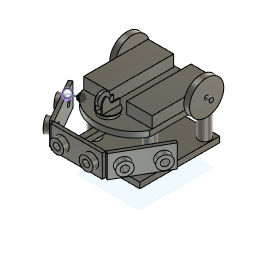
Chassis v4 (Autodesk Fusion 360 design; units mm, degrees)
Autodesk Fusion 360 part; units mm, degrees
sketch "Sketch1" plane through (0, 0, 0) normal (1, 0, 0) x (0, 1, 0)
  line L0 (30, -30) -> (-30, -30)
  line L1 (-30, -30) -> (-30, 30)
  line L2 (30, 30) -> (30, -30)
  line L3 (30, -30) -> (-30, 30) construction
  line L4 (-30, -30) -> (30, 30) construction
  arc A0 (30, 30) -> (-30, 30) centre (0, 12.4031) ccw
  dimension "d1" = 60
  dimension "d2" = 60
  constraint horizontal L0
  constraint perpendicular L0 L1
  constraint parallel L1 L2
  constraint coincident L3 origin
  constraint coincident L4 origin
  measures "d1" distance of L1.end L2.start
  measures "d2" distance of L0.end L1.end
extrude "Extrude1" add sketch "Sketch1" along normal blind 5 makes body 1
move_body "Move1" bodies 1 to x (0, 0, 1) y (-1, 0, 0) z (0, -1, 0) at (-30, -60, 0)
sketch "Sketch2" plane through (0, 0, 0) normal (0, 0, -1) x (1, 0, 0)
  line L0 (-60, 90) -> (-60, 30)
  line L1 (-60, 30) -> (0, 30)
  line L2 (0, 30) -> (0, 90)
  arc A0 (0, 90) -> (-60, 90) centre (-30, 72.4031) ccw
  circle A1 centre (-5.7984, 36.1081) radius 5
  line L3 (-30, 27.885) -> (-30, 109.1678) construction
  line L4 (-30, 27.885) -> (-30, 109.1678) construction
  circle A2 centre (-54.2016, 36.1081) radius 5
  line L5 (25, 60) -> (-75, 60) construction
  line L6 (25, 60) -> (-75, 60) construction
  circle A3 centre (-5.7984, 83.8919) radius 5
  circle A4 centre (-54.2016, 83.8919) radius 5
  dimension "d5" = 10
  constraint perpendicular L1 L3
  constraint symmetric A1 L3 A2
  constraint symmetric L4.start L3 L3.start
  constraint symmetric L4.end L3 L3.end
  constraint perpendicular L0 L5
  constraint symmetric A1 L5 A3
  constraint symmetric A2 L5 A4
  constraint symmetric L6.start L5 L5.start
  constraint symmetric L6.end L5 L5.end
  measures "d5" diameter of A1
extrude "Extrude2" add sketch "Sketch2" along normal blind 30 contours A1 | A2 | A3 | A4 bodies 1
ref_plane "WorkPlane1" through (-30, -68.5916, -50) normal (0, 0, -1) x (1, 0, 0)
sketch "Sketch3" plane through (-30, -68.5916, -50) normal (0, 0, -1) x (-1, 0, 0)
  line L0 (-30, -21.4084) -> (-30, 38.5916)
  line L1 (30, 38.5916) -> (30, -21.4084)
  line L2 (-30, -30) -> (-30, 40)
  line L3 (30, 40) -> (-30, 40)
  line L4 (-30, -30) -> (30, -30)
  line L5 (30, -30) -> (30, 40)
  point P0 (-30, 38.5916)
  point P1 (30, 38.5916)
  point P2 (30, -21.4084)
  point P3 (-30, -21.4084)
  dimension "d10" = 60
  dimension "d11" = 70
  constraint vertical L0
  constraint vertical L1
  constraint coincident P0 L0.end
  constraint coincident P2 L1.end
  constraint perpendicular L2 L3
  constraint perpendicular L2 L4
  constraint perpendicular L3 L5
  measures "d10" distance of P2 P3
  measures "d11" distance of L2.start L2.end
extrude "Extrude3" add sketch "Sketch3" along normal blind 5 bodies 1 makes body 2
sketch "Sketch4" plane through (0, 0, 5) normal (0, 0, 1) x (-1, 0, 0)
  line L0 (60, 30) -> (60, 90)
  arc A0 (60, 90) -> (0, 90) centre (30, 72.4031) ccw
  line L1 (0, 90) -> (0, 30)
  line L2 (0, 30) -> (60, 30)
  line L3 (0, 87.7947) -> (22.4, 87.7947)
  line L4 (22.4, 87.7947) -> (22.4, 31.2947)
  line L5 (22.4, 31.2947) -> (0, 31.2947)
  line L6 (0, 31.2947) -> (0, 87.7947)
  line L7 (30, 125) -> (30, 18.4359) construction
  line L8 (30, 125) -> (30, 18.4359) construction
  line L9 (60, 87.7947) -> (37.6, 87.7947)
  line L10 (37.6, 87.7947) -> (37.6, 31.2947)
  line L11 (37.6, 31.2947) -> (60, 31.2947)
  line L12 (60, 31.2947) -> (60, 87.7947)
  dimension "d14" = 22.4
  dimension "d15" = 56.5
  constraint horizontal L3
  constraint vertical L4
  constraint horizontal L5
  constraint vertical L6
  constraint coincident L1 L3.start
  constraint perpendicular L2 L7
  constraint symmetric L3.start L7 L9.start
  constraint symmetric L3.end L7 L9.end
  constraint symmetric L4.end L7 L10.end
  constraint symmetric L5.end L7 L11.end
  constraint symmetric L8.start L7 L7.start
  constraint symmetric L8.end L7 L7.end
  measures "d14" distance of L3.start L3.end
  measures "d15" distance of L3.start L5.end
extrude "Extrude4" add sketch "Sketch4" along normal blind 10 separate body contours L0 L9 L10 L11 L12 | L1 L3 L4 L5 L6 makes body 3 at (-45.0667, -68.9614, 5) makes body 4 at (-7.4667, -50.1281, 5)
sketch "Sketch5" plane through (-60, 0, 0) normal (-1, 0, 0) x (0, -1, 0)
  line L0 (31.2947, 5) -> (87.7947, 5)
  line L1 (87.7947, 5) -> (87.7947, 15)
  line L2 (87.7947, 15) -> (31.2947, 15)
  line L3 (31.2947, 15) -> (31.2947, 5)
  line L4 (44.9519, 15) -> (44.9519, 5) construction
  circle A0 centre (44.9519, 10) radius 1.85
  dimension "d18" = 3.7
  constraint coincident L2 L4.start
  constraint coincident L0 L4.end
  constraint perpendicular L0 L4
  constraint midpoint L4 A0.centre
  measures "d18" diameter of A0
extrude "Extrude5" add sketch "Sketch5" along normal blind 9.1 contours A0 bodies 3
sketch "Sketch6" plane through (0, 0, 0) normal (1, 0, 0) x (0, 1, 0)
  line L0 (-87.7947, 5) -> (-31.2947, 5)
  line L1 (-31.2947, 5) -> (-31.2947, 15)
  line L2 (-31.2947, 15) -> (-87.7947, 15)
  line L3 (-87.7947, 15) -> (-87.7947, 5)
  circle A0 centre (-44.9519, 10) radius 1.85
  circle A1 centre (-44.9519, 10) radius 1.85
  constraint concentric A0 A1
extrude "Extrude6" add sketch "Sketch6" along normal blind 9.1 contours A0 A1 bodies 4
sketch "Sketch7" plane through (-60, 0, 0) normal (-1, 0, 0) x (0, -1, 0)
  circle A0 centre (44.9519, 10) radius 1.85
  line L0 (31.2947, 5) -> (87.7947, 5)
  line L1 (87.7947, 5) -> (87.7947, 15)
  line L2 (87.7947, 15) -> (31.2947, 15)
  line L3 (31.2947, 15) -> (31.2947, 5)
  circle A1 centre (44.9519, 10) radius 15
  dimension "d23" = 30
  constraint concentric A0 A1
  measures "d23" diameter of A1
extrude "Extrude7" add sketch "Sketch7" along normal blind 5 separate body contours L0 L2 L3 A1 | L0 L2 L3 A1 makes body 5
sketch "Sketch8" plane through (0, 0, 0) normal (1, 0, 0) x (0, 1, 0)
  circle A0 centre (-44.9519, 10) radius 1.85
  line L0 (-87.7947, 5) -> (-31.2947, 5)
  line L1 (-31.2947, 5) -> (-31.2947, 15)
  line L2 (-31.2947, 15) -> (-87.7947, 15)
  line L3 (-87.7947, 15) -> (-87.7947, 5)
  circle A1 centre (-44.9519, 10) radius 1.85
  circle A2 centre (-44.9519, 10) radius 15
  circle A3 centre (-44.9519, 10) radius 15
  constraint concentric A1 A3
extrude "Extrude8" add sketch "Sketch8" along normal blind 5 separate body contours L0 L1 L2 A2 A3 | L0 L1 L2 A2 A3 makes body 6
sketch "Sketch9" plane through (0, 0, 5) normal (0, 0, 1) x (-1, 0, 0)
  line L0 (60, 30) -> (60, 90)
  arc A0 (60, 90) -> (0, 90) centre (30, 72.4031) ccw
  line L1 (0, 90) -> (0, 30)
  line L2 (0, 30) -> (60, 30)
  line L3 (60, 90) -> (0, 90) construction
  line L4 (37.6, 90) -> (22, 90)
  line L5 (22, 90) -> (22, 104)
  line L6 (22, 104) -> (37.6, 104)
  line L7 (37.6, 104) -> (37.6, 90)
  line L8 (29.8, 90) -> (29.8, 103) construction
  circle A1 centre (29.8, 96.5) radius 3.8567
  point P0 (37.6, 87.7947)
  point P1 (22.4, 87.7947)
  point P2 (60, 90)
  point P3 (0, 90)
  constraint coincident P2 L0.end
  constraint coincident P3 A0.end
  constraint horizontal L4
  constraint vertical L5
  constraint horizontal L6
  constraint vertical L7
  constraint coincident L3 L4.start
  constraint midpoint L4 L8.start
  constraint perpendicular L3 L8
  constraint midpoint L8 A1.centre
extrude "Extrude9" add sketch "Sketch9" along normal blind 2 contours A1 bodies 1 2
sketch "Sketch14" plane through (0, 0, 0) normal (1, 0, 0) x (0, 1, 0)
  line L0 (-99.4, 14.3, -27) -> (-104.6, 14.3, -27)
  line L1 (-104.6, 14.3, -27) -> (-104.6, 22.3, -27)
  spline S0 degree 5 poles (-104.6, 22.3, -27) (-104.4812, 22.5487, -27) (-104.241, 23.0305, -27) (-103.8731, 23.7067, -27) (-103.3671, 24.5146, -27) (-102.7085, 25.3544, -27) (-102.0235, 25.9895, -27) (-101.3124, 26.3564, -27) (-100.5764, 26.3524, -27) (-99.8191, 25.8256, -27) (-99.084, 24.8415, -27) (-98.4247, 23.5629, -27) (-97.8903, 22.2148, -27) (-97.5026, 21.0151, -27) (-97.2403, 20.1286, -27) (-97.0075, 19.5905, -27) (-96.7307, 19.3846, -27) (-96.4147, 19.3154, -27) (-96.1476, 19.3, -27) (-96, 19.3, -27) knots 0 0 0 0 0 0 0.06666667 0.13333333 0.2 0.26666667 0.33333333 0.4 0.46666667 0.53333333 0.6 0.66666667 0.73333333 0.8 0.86666667 0.93333333 1 1 1 1 1 1
  line L2 (-102, 26.3, -27) -> (-100, 26.3, -27)
  line L3 (-98, 19.3, -27) -> (-94, 19.3, -27)
  line L4 (-96, 19.3, -27) -> (-89, 19.3, -27)
  line L5 (-89, 19.3, -27) -> (-89, 14.3, -27)
  line L6 (-89, 14.3, -27) -> (-99.4, 14.3, -27)
  circle A0 through (-95.5, 23.3, -27) (-103.75, 28.0631, -27) (-103.75, 18.5369, -27)
  circle A1 through (-99.5, 23.3, -27) (-101.75, 24.599, -27) (-101.75, 22.001, -27)
  point P0 (-101, 26.3)
  point P1 (-97.4208, 20.7375)
  dimension "d47" = 8
  dimension "d48" = 11
  dimension "d50" = 3
extrude "Extrude17" add sketch "Sketch14" against normal blind 1 separate body contours L0 L1 L3 L4 L5 L6 A0 | L1 S0 A0 | S0 L3 A0 in plane through (-27, 0, 0) normal (1, 0, 0) picked at (-27, -103.7117, 21.1897) makes body 7
ref_plane "WorkPlane4" through (-32.6, -96.8, 20.3063) normal (1, 0, 0) x (0, 1, 0)
sketch "Sketch15" plane through (-32.6, -96.8, 20.3063) normal (1, 0, 0) x (0, 1, 0)
  circle A0 centre (-4.2, 2.9937) radius 1.5
  line L0 (7.8, -1.0063) -> (7.8, -6.0063)
  line L1 (7.8, -6.0063) -> (-2.6, -6.0063)
  line L2 (-2.6, -6.0063) -> (-7.8, -6.0063)
  line L3 (-7.8, -6.0063) -> (-7.8, 1.9937)
  spline S0 degree 5 poles (-7.8, 1.9937) (-7.6812, 2.2423) (-7.441, 2.7242) (-7.0731, 3.4004) (-6.5671, 4.2082) (-5.9085, 5.0481) (-5.2235, 5.6831) (-4.5124, 6.0501) (-3.7764, 6.0461) (-3.0191, 5.5193) (-2.284, 4.5351) (-1.6247, 3.2566) (-1.0903, 1.9085) (-0.7026, 0.7088) (-0.4403, -0.1778) (-0.2075, -0.7158) (0.0693, -0.9218) (0.3853, -0.991) (0.6524, -1.0063) (0.8, -1.0063) knots 0 0 0 0 0 0 0.066667 0.133333 0.2 0.266667 0.333333 0.4 0.466667 0.533333 0.6 0.666667 0.733333 0.8 0.866667 0.933333 1 1 1 1 1 1
  line L4 (0.8, -1.0063) -> (7.8, -1.0063)
extrude "Extrude18" add sketch "Sketch15" against normal blind 1 separate body makes body 8
extrude "Extrude19" add sketch "Sketch14" against normal blind 6.6 contours A1 in plane through (-27, 0, 0) normal (1, 0, 0) bodies 7 8
ref_plane "WorkPlane5" through (-30.3, -96.8, 20.3063) normal (-1, 0, 0) x (0, -1, 0)
sketch "Sketch16" plane through (-30.3, -96.8, 20.3063) normal (-1, 0, 0) x (0, -1, 0)
  circle A0 centre (4.2, 2.9937) radius 5.5
  circle A1 centre (4.2, 2.9937) radius 5.5
  constraint concentric A0 A1
extrude "Extrude20" add sketch "Sketch16" along normal mid plane 2.5 separate body makes body 9
ref_plane "WorkPlane6" through (-29.8, -96.5, 14.3) normal (0, 0, 1) x (-1, 0, 0)
sketch "Sketch17" plane through (-29.8, -96.5, 14.3) normal (0, 0, 1) x (1, 0, 0)
  circle A0 centre (0, 0) radius 8.6023
  constraint coincident A0.centre origin
extrude "Extrude21" add sketch "Sketch17" against normal blind 1 separate body makes body 10
fillet "Fillet1" radius 0.5 1 edges at (-37.8202, -93.3893, 13.3) on bodies 10
sketch "Sketch18" plane through (0, 0, 7) normal (0, 0, 1) x (-1, 0, 0)
  circle A0 centre (29.8, 96.5) radius 3.8567
  circle A1 centre (29.8, 96.5) radius 8.6023
  circle A2 centre (29.8, 96.5) radius 7.8023
  dimension "d65" = -0.8
extrude "Extrude22" add sketch "Sketch18" along normal blind 2.5 contours A0 | A2 bodies 2 1
move_body "Move5" bodies 10 9 7 to x (1, 0, 0) y (0, 1, 0) z (0, 0, 1) at (0, 0, -3.3)
move_body "Move6" bodies 9 7 10 to x (1, 0, 0) y (0, 1, 0) z (0, 0, 1) at (0, 0, -0.5)
sketch "Sketch19" plane through (0, 0, 0) normal (1, 0, 0) x (0, 1, 0)
  line L0 (-180, 0) -> (-135, 0)
  line L1 (-135, 0) -> (-135, -20)
  line L2 (-135, -20) -> (-180, -20)
  line L3 (-180, -20) -> (-180, 0)
  dimension "d68" = 45
  dimension "d69" = 20
  constraint horizontal L0
  constraint vertical L1
  constraint horizontal L2
  constraint vertical L3
  measures "d68" distance of L0.start L0.end
  measures "d69" distance of L0.start L2.end
extrude "Extrude23" add sketch "Sketch19" along normal blind 3 separate body makes body 11
sketch "Sketch20" plane through (3, 0, 0) normal (1, 0, 0) x (0, 1, 0)
  line L0 (-180, -20) -> (-135, -20)
  line L1 (-135, -20) -> (-135, 0)
  line L2 (-135, 0) -> (-180, 0)
  line L3 (-180, 0) -> (-180, -20)
  circle A0 centre (-144.2379, -10) radius 6
  circle A1 centre (-170, -10) radius 6
  circle A2 centre (-144.2379, -10) radius 3
  circle A3 centre (-170, -10) radius 3
  dimension "d72" = 12
  dimension "d73" = 12
  dimension "d74" = 6
  dimension "d75" = 6
  constraint concentric A0 A2
  constraint concentric A1 A3
  measures "d72" diameter of A0
  measures "d73" diameter of A1
  measures "d74" diameter of A2
  measures "d75" diameter of A3
extrude "Extrude24" cut sketch "Sketch20" against normal through all contours A2 | A3 bodies 11
extrude "Extrude25" add sketch "Sketch20" along normal blind 5 contours A0 | A1 bodies 11
move_body "Move7" bodies 11 to x (0.000333, -0.999971, -0.007596) y (1, 0.00033, 0.000333) z (-0.00033, -0.007596, 0.999971) at (126.5286, -97.5558, 0.672)
sketch "Sketch21" plane through (0, 0, -55) normal (0, 0, -1) x (1, 0, 0)
  line L0 (0, 98.5916) -> (-60, 98.5916)
  line L1 (-60, 98.5916) -> (-60, 28.5916)
  line L2 (-60, 28.5916) -> (0, 28.5916)
  line L3 (0, 28.5916) -> (0, 98.5916)
  line L4 (-2.0421, 32.2156) -> (-57.0421, 32.2156)
  line L5 (-57.0421, 32.2156) -> (-57.0421, 97.2156)
  line L6 (-57.0421, 97.2156) -> (-2.0421, 97.2156)
  line L7 (-2.0421, 97.2156) -> (-2.0421, 32.2156)
  line L8 (-2.0421, 32.2156) -> (-57.0421, 97.2156) construction
  line L9 (-57.0421, 32.2156) -> (-2.0421, 97.2156) construction
  point P0 (-29.5421, 64.7156)
  dimension "d79" = 55
  dimension "d80" = 65
  constraint horizontal L4
  constraint perpendicular L4 L5
  constraint parallel L4 L6
  constraint parallel L5 L7
  constraint coincident L8 P0
  constraint coincident L9 P0
  measures "d79" distance of L5.end L6.end
  measures "d80" distance of L4.end L5.end
extrude "Extrude26" cut sketch "Sketch21" against normal blind 2 contours L4 L5 L6 L7 bodies 1 2
sketch "Sketch22" plane through (0, 0, 0) normal (0, 0, -1) x (1, 0, 0)
  circle A0 centre (-54.2016, 83.8919) radius 5
  circle A1 centre (-5.7984, 83.8919) radius 5
  circle A2 centre (-54.2016, 36.1081) radius 5
  circle A3 centre (-5.7984, 36.1081) radius 5
  line L0 (-60, 90) -> (-60, 30)
  line L1 (-60, 30) -> (0, 30)
  line L2 (0, 30) -> (0, 90)
  arc A4 (0, 90) -> (-60, 90) centre (-30, 72.4031) ccw
  line L3 (-12, 47) -> (-48, 47)
  line L4 (-48, 47) -> (-48, 93)
  line L5 (-48, 93) -> (-12, 93)
  line L6 (-12, 93) -> (-12, 47)
  line L7 (-12, 47) -> (-48, 93) construction
  line L8 (-48, 47) -> (-12, 93) construction
  point P0 (-30, 70)
  dimension "d83" = 36
  dimension "d84" = 46
  constraint horizontal L3
  constraint perpendicular L3 L4
  constraint parallel L3 L5
  constraint parallel L4 L6
  constraint coincident L7 P0
  constraint coincident L8 P0
  measures "d83" distance of L4.end L5.end
  measures "d84" distance of L3.end L4.end
extrude "Extrude27" cut sketch "Sketch22" against normal blind 2 contours L3 L4 L5 L6 bodies 1 2
copy_body "CopyPasteBodies1" bodies 11 makes body 12
move_body "Move8" bodies 12 to x (1, 0, 0) y (0, 1, 0) z (0, 0, 1) at (0, -125.493, -71.5311)
copy_body "CopyPasteBodies2" bodies 11 makes body 13
move_body "Move9" bodies 13 to x (1, 0, 0) y (0, 1, 0) z (0, 0, 1) at (0, -96.6237, -76.8345)
move_body "Move10" bodies 11 to x (1, 0, 0) y (0, 1, 0) z (0, 0, 1) at (0, -53, 0)
sketch "Sketch23" plane through (0, 0, 0) normal (0, 0, -1) x (1, 0, 0)
  line L0 (-48, 47) -> (-48, 93)
  line L1 (-48, 93) -> (-12, 93)
  line L2 (-12, 93) -> (-12, 47)
  line L3 (-12, 47) -> (-48, 47)
  circle A0 centre (-54.2016, 83.8919) radius 5
  circle A1 centre (-5.7984, 83.8919) radius 5
  circle A2 centre (-54.2016, 36.1081) radius 5
  circle A3 centre (-5.7984, 36.1081) radius 5
  line L4 (-60, 90) -> (-60, 30)
  line L5 (-60, 30) -> (0, 30)
  line L6 (0, 30) -> (0, 90)
  arc A4 (0, 90) -> (-60, 90) centre (-30, 72.4031) ccw
  line L7 (-27, 101) -> (-32, 101)
  line L8 (-32, 101) -> (-32, 122)
  line L9 (-32, 122) -> (-27, 122)
  line L10 (-27, 122) -> (-27, 101)
  constraint horizontal L7
  constraint vertical L8
  constraint horizontal L9
  constraint vertical L10
extrude "Extrude28" add sketch "Sketch23" along normal blind 5 contours A4 L8 L9 L10 | A4 L7 L8 L10 bodies 2 1
move_body "Move11" bodies 11 to x (1, 0, 0) y (0, 1, 0) z (0, 0, 1) at (0.5, 30, 0)
move_body "Move12" bodies 12 to x (0.5, -0.866025, 0) y (0.866025, 0.5, 0) z (0, 0, 1) at (76.5915, -6.6381, 71.5)
move_body "Move13" bodies 12 to x (1, 0, 0) y (0, 1, 0) z (0, 0, 1) at (70, -8, 0)
move_body "Move14" bodies 13 to x (0.5, 0.866025, 0) y (-0.866025, 0.5, 0) z (0, 0, 1) at (-149.3351, 23.0399, 76.9)
move_body "Move15" bodies 12 to x (1, 0, 0) y (0, 1, 0) z (0, 0, 1) at (-3, 0, 0)
move_body "Move16" bodies 12 to x (1, 0, 0) y (0, 1, 0) z (0, 0, 1) at (0.6, -1.7, 0)
sketch "Sketch25" plane through (0, 0, 0) normal (0, 0, -1) x (1, 0, 0)
  line L0 (-32, 101) -> (-32, 107.1256)
  arc A0 (-32, 107.1256) -> (-60, 90) centre (-30, 72.4031) ccw
  line L1 (-60, 90) -> (-60, 30)
  line L2 (-60, 30) -> (0, 30)
  line L3 (0, 30) -> (0, 90)
  arc A1 (0, 90) -> (-27, 107.0535) centre (-30, 72.4031) ccw
  line L4 (-27, 107.0535) -> (-27, 101)
  line L5 (-27, 101) -> (-32, 101)
  line L6 (-48, 47) -> (-48, 93)
  line L7 (-48, 93) -> (-12, 93)
  line L8 (-12, 93) -> (-12, 47)
  line L9 (-12, 47) -> (-48, 47)
  circle A2 centre (-54.2016, 83.8919) radius 5
  circle A3 centre (-5.7984, 83.8919) radius 5
  circle A4 centre (-54.2016, 36.1081) radius 5
  circle A5 centre (-5.7984, 36.1081) radius 5
  line L10 (-60, 90) -> (-69.3, 92.7)
  constraint coincident A0.end L1.start
sketch "Sketch26" plane through (-92.131, -53.2328, -0.8083) normal (0.865834, 0.500274, 0.007596) x (-0.500288, 0.865859, 0)
  circle A0 centre (-68.5037, -8.5988) radius 3
  circle A1 centre (-42.7415, -8.6074) radius 3
  line L0 (-77.7449, -18.5957) -> (-32.7449, -18.6107)
  line L1 (-32.7449, -18.6107) -> (-32.7382, 1.3893)
  line L2 (-32.7382, 1.3893) -> (-77.7382, 1.4042)
  line L3 (-77.7382, 1.4042) -> (-77.7449, -18.5957)
  line L4 (-47.91, 0.7366) -> (-45.5951, 0.8081)
  circle A2 centre (-45.94, 0.83) radius 0.75
  point P0 (-45.5951, 0.8081)
  point P1 (-47.91, 0.7366)
  dimension "d89" = 1.5
  measures "d89" diameter of A2
sweep "Sweep1" add profiles "Sketch26" path "Sketch25" along L10 section 1 contours L2 A2 | L2 A2 bodies 12
extrude "Extrude29" add 1 faces at (-59.9517, -90.1451, 0.1596) along direction (0.865834, 0.500274, 0.007596) blind 0.2 on bodies 12 bodies 12 2 1
sketch "Sketch28" plane through (0, 0, 0) normal (0, 0, -1) x (1, 0, 0)
  line L0 (0, 90) -> (7.35, 94.1)
sketch "Sketch29" plane through (46.2086, -26.658, -0.4052) normal (-0.866167, 0.499697, 0.007596) x (-0.499712, -0.866192, 0)
  circle A0 centre (72.4381, -8.9053) radius 3
  circle A1 centre (98.2002, -8.9139) radius 3
  line L0 (63.1969, -18.9022) -> (108.1969, -18.9172)
  line L1 (108.1969, -18.9172) -> (108.2035, 1.0828)
  line L2 (108.2035, 1.0828) -> (63.2035, 1.0978)
  line L3 (63.2035, 1.0978) -> (63.1969, -18.9022)
  circle A2 centre (77.9573, 0.3416) radius 0.75
  point P0 (77.9573, 0.3416)
  dimension "d98" = 1.5
  constraint coincident P0 A2.centre
  measures "d98" diameter of A2
sweep "Sweep2" add profiles "Sketch29" path "Sketch28" along L0 section 1 contours A2 bodies 13
extrude "Extrude30" add 1 faces at (-0.1364, -90.2397, 0.2203) along direction (-0.866167, 0.499697, 0.007596) blind 0.2 on bodies 13 bodies 13 2 12
sketch "Sketch30" plane through (0, 0, -53) normal (0, 0, -1) x (1, 0, 0)
  line L0 (-2.0421, 97.2156) -> (-57.0421, 97.2156)
  line L1 (-57.0421, 97.2156) -> (-57.0421, 32.2156)
  line L2 (-57.0421, 32.2156) -> (-2.0421, 32.2156)
  line L3 (-2.0421, 32.2156) -> (-2.0421, 97.2156)
move_body "Move17" bodies 2 to x (1, 0, 0) y (0, 1, 0) z (0, 0, 1) at (0, 0, 20)
